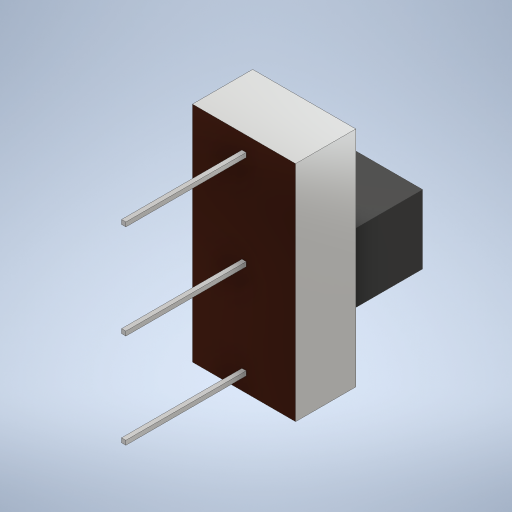
# Autodesk Inventor part: switch small
Saved by Autodesk Inventor 2023 (Build 270158000, 158)
## iProperties
Created: 2018-07-03
Part Number: switch small
Material: Generic
Document SubType Name: Modeling
Designer: adams
Density: 1 g/cm^3
Appearance: Aluminum - Polished
Author: adams
Autodesk Inventor part; units mm, degrees
ref_plane "YZ Plane" through (0, 0, 0) normal (1, 0, 0) x (0, 1, 0)
ref_plane "XZ Plane" through (0, 0, 0) normal (0, 1, 0) x (-1, 0, 0)
ref_plane "XY Plane" through (0, 0, 0) normal (0, 0, 1) x (1, 0, 0)
sketch "Sketch1" plane through (0, 0, 0) normal (0, 1, 0) x (-1, 0, 0)
  line L0 (0, 0) -> (-6, 0)
  line L1 (-6, 0) -> (-6, -13)
  line L2 (-6, -13) -> (0, -13)
  line L3 (0, -13) -> (0, 0)
  dimension "d0" = 6
  dimension "d1" = 13
  constraints: 8 end point, 2 parallel, 1 horizontal, 1 perpendicular
  measures "d0" distance of L2.end L1.end
  measures "d1" distance of L1.end L0.end
extrude "Extrusion1" add sketch "Sketch1" along normal blind 3.5
sketch "Sketch2" plane through (0, 3.5, 0) normal (0, 1, 0) x (1, 0, 0)
  line L0 (0, 13) -> (0, 0) projected
  line L1 (6, 0) -> (6, 13) projected
  line L2 (0, 0) -> (6, 0)
  line L3 (6, 0) -> (6, 13)
  line L4 (6, 13) -> (0, 13)
  line L5 (0, 13) -> (0, 0)
  line L6 (3, 0) -> (6.25, 0) construction
  line L7 (2, 3) -> (1.5, 3)
  line L8 (1.5, 3) -> (1, 3)
  line L9 (1.5, 3) -> (2, 3) construction
  line L10 (2, 3) -> (5, 3)
  line L11 (2, 3) -> (5, 3) construction
  line L12 (5, 3) -> (5, 10)
  line L13 (5, 10) -> (1, 10)
  line L14 (1, 10) -> (1, 3)
  line L15 (1, 3) -> (5, 3)
  line L16 (5, 3) -> (5, 10)
  line L17 (5, 10) -> (1, 10)
  line L18 (1, 10) -> (1, 3)
  dimension "d41" = 3
  dimension "d42" = 1
  dimension "d44" = 1
  dimension "d45" = 3
  constraints: 34 end point, 7 horizontal, 5 perpendicular, 4 parallel, 3 collinear, 1 midpoint
  measures "d41" distance between parallel lines of L4 L13
  measures "d42" distance between parallel lines of L0 L14
  measures "d44" distance between parallel lines of L1 L12
  measures "d45" distance between parallel lines of L10 L2
extrude "Extrusion3" cut sketch "Sketch2" against normal blind 0.11 contours L7 L8 L14 L13 L12 L10
sketch "Sketch3" plane through (0, 3.39, 0) normal (0, 1, 0) x (1, 0, 0)
  line L0 (1, 3) -> (1, 10) projected
  line L1 (1, 10) -> (5, 10)
  line L2 (5, 10) -> (5, 6)
  line L3 (5, 6) -> (1, 6)
  line L4 (1, 6) -> (1, 10)
  point P0 (0, 0)
  dimension "d20" = 4
  dimension "d21" = 4
  constraints: 8 end point, 2 parallel, 1 horizontal, 1 perpendicular
  measures "d20" distance of L2.end L3.end
  measures "d21" distance of L1.end L2.end
extrude "Extrusion4" add sketch "Sketch3" along normal blind 5
sketch "Sketch4" plane through (0, 0, 0) normal (0, -1, 0) x (1, 0, 0)
  line L0 (0, 0) -> (6, 0) projected
  line L1 (3, 0) -> (3, -1) construction
  line L2 (3, 0) -> (4, 0) construction
  line L3 (2.875, -1.125) -> (3.125, -1.125)
  line L4 (3.125, -1.125) -> (3.125, -0.875)
  line L5 (3.125, -0.875) -> (2.875, -0.875)
  line L6 (2.875, -0.875) -> (2.875, -1.125)
  line L7 (2.875, -1.125) -> (3.125, -0.875) construction
  line L8 (3.125, -1.125) -> (2.875, -0.875) construction
  line L9 (6, -13) -> (0, -13) projected
  line L10 (3, -13) -> (3, -12) construction
  line L11 (3, -13) -> (4, -13) construction
  line L12 (2.875, -12.125) -> (3.125, -12.125)
  line L13 (3.125, -12.125) -> (3.125, -11.875)
  line L14 (3.125, -11.875) -> (2.875, -11.875)
  line L15 (2.875, -11.875) -> (2.875, -12.125)
  line L16 (2.875, -12.125) -> (3.125, -11.875) construction
  line L17 (3.125, -12.125) -> (2.875, -11.875) construction
  line L18 (3, -0.875) -> (3, -6.5) construction
  line L19 (3, -0.875) -> (8.625, -0.875) construction
  line L20 (2.875, -6.625) -> (3.125, -6.625)
  line L21 (3.125, -6.625) -> (3.125, -6.375)
  line L22 (3.125, -6.375) -> (2.875, -6.375)
  line L23 (2.875, -6.375) -> (2.875, -6.625)
  line L24 (2.875, -6.625) -> (3.125, -6.375) construction
  line L25 (3.125, -6.625) -> (2.875, -6.375) construction
  point P0 (3, -6.5)
  dimension "d24" = 1
  dimension "d25" = 90
  dimension "d26" = 0.25
  dimension "d27" = 0.25
  dimension "d28" = 1
  dimension "d29" = 90
  dimension "d30" = 0.25
  dimension "d31" = 0.25
  dimension "d33" = 90
  dimension "d34" = 0.25
  dimension "d35" = 0.25
  dimension "d39" = 5.5
  dimension "d40" = 5.5
  constraints: 48 end point, 10 midpoint, 6 horizontal, 6 parallel, 6 perpendicular, 3 vertical
  measures "d24" distance of L1.start L1.end
  measures "d25" angle of L1 L2
  measures "d26" distance of L5.end L4.end
  measures "d27" distance of L4.end L3.end
  measures "d28" distance of L10.start L10.end
  measures "d29" angle of L11 L10
  measures "d30" distance of L14.end L13.end
  measures "d31" distance of L13.end L12.end
  measures "d33" angle of L18 L19
  measures "d34" distance of L22.end L21.end
  measures "d35" distance of L21.end L20.end
  measures "d39" distance between parallel lines of L22 L5
  measures "d40" distance between parallel lines of L12 L20
extrude "Extrusion5" add sketch "Sketch4" along normal blind 7
equation "\"d41\" = d5"
equation "\"d44\" = d42"
equation "\"d45\" = d41"
equation "\"d21\" = d20"
equation "\"d24\" = d28"
equation "\"d5\" = 3"
body "Solid1"
